Autodesk Fusion 360 part; units mm, degrees
note: some values were not read from the file. Set by a fixed rule: which face or edge a step refers to.
(part 3 of 3)
sketch "スケッチ8" plane through (0, 0, 2) normal (0, 0, 1) x (-1, 0, 0)
  line L0 (-93, 22) -> (-93, 18)
  line L1 (-93, 18) -> (-97, 18)
  line L2 (-97, 18) -> (-97, 22)
  line L3 (-97, 22) -> (-93, 22)
  line L4 (-13, 22) -> (-13, 18)
  line L5 (-13, 18) -> (-17, 18)
  line L6 (-17, 18) -> (-17, 22)
  line L7 (-17, 22) -> (-13, 22)
  line L8 (-47, -18) -> (-43, -18)
  line L9 (-43, -18) -> (-43, -22)
  line L10 (-43, -22) -> (-47, -22)
  line L11 (-47, -22) -> (-47, -18)
  line L12 (33, -18) -> (37, -18)
  line L13 (37, -18) -> (37, -22)
  line L14 (37, -22) -> (33, -22)
  line L15 (33, -22) -> (33, -18)
  arc A0 (-93.85, -22.9326) -> (-96.15, -22.9326) centre (-95, -20) ccw
  line L16 (-93.85, -22.9326) -> (-93.85, -24)
  line L17 (-93.85, -24) -> (-92, -24)
  line L18 (-92, -24) -> (-92, -27)
  line L19 (-92, -27) -> (-98, -27)
  line L20 (-98, -27) -> (-98, -24)
  line L21 (-98, -24) -> (-96.15, -24)
  line L22 (-96.15, -24) -> (-96.15, -22.9326)
  arc A1 (-73.85, -22.9326) -> (-76.15, -22.9326) centre (-75, -20) ccw
  line L23 (-73.85, -22.9326) -> (-73.85, -24)
  line L24 (-73.85, -24) -> (-72, -24)
  line L25 (-72, -24) -> (-72, -27)
  line L26 (-72, -27) -> (-78, -27)
  line L27 (-78, -27) -> (-78, -24)
  line L28 (-78, -24) -> (-76.15, -24)
  line L29 (-76.15, -24) -> (-76.15, -22.9326)
  arc A2 (-53.85, -22.9326) -> (-56.15, -22.9326) centre (-55, -20) ccw
  line L30 (-53.85, -22.9326) -> (-53.85, -24)
  line L31 (-53.85, -24) -> (-52, -24)
  line L32 (-52, -24) -> (-52, -27)
  line L33 (-52, -27) -> (-58, -27)
  line L34 (-58, -27) -> (-58, -24)
  line L35 (-58, -24) -> (-56.15, -24)
  line L36 (-56.15, -24) -> (-56.15, -22.9326)
  arc A3 (-33.85, -22.9326) -> (-36.15, -22.9326) centre (-35, -20) ccw
  line L37 (-33.85, -22.9326) -> (-33.85, -24)
  line L38 (-33.85, -24) -> (-32, -24)
  line L39 (-32, -24) -> (-32, -27)
  line L40 (-32, -27) -> (-38, -27)
  line L41 (-38, -27) -> (-38, -24)
  line L42 (-38, -24) -> (-36.15, -24)
  line L43 (-36.15, -24) -> (-36.15, -22.9326)
  arc A4 (-13.85, -22.9326) -> (-16.15, -22.9326) centre (-15, -20) ccw
  line L44 (-13.85, -22.9326) -> (-13.85, -24)
  line L45 (-13.85, -24) -> (-12, -24)
  line L46 (-12, -24) -> (-12, -27)
  line L47 (-12, -27) -> (-18, -27)
  line L48 (-18, -27) -> (-18, -24)
  line L49 (-18, -24) -> (-16.15, -24)
  line L50 (-16.15, -24) -> (-16.15, -22.9326)
  arc A5 (6.15, -22.9326) -> (3.85, -22.9326) centre (5, -20) ccw
  line L51 (6.15, -22.9326) -> (6.15, -24)
  line L52 (6.15, -24) -> (8, -24)
  line L53 (8, -24) -> (8, -27)
  line L54 (8, -27) -> (2, -27)
  line L55 (2, -27) -> (2, -24)
  line L56 (2, -24) -> (3.85, -24)
  line L57 (3.85, -24) -> (3.85, -22.9326)
  arc A6 (-18.85, -2.9326) -> (-21.15, -2.9326) centre (-20, 0) ccw
  line L58 (-18.85, -2.9326) -> (-18.85, -4)
  line L59 (-18.85, -4) -> (-17, -4)
  line L60 (-17, -4) -> (-17, -7)
  line L61 (-17, -7) -> (-23, -7)
  line L62 (-23, -7) -> (-23, -4)
  line L63 (-23, -4) -> (-21.15, -4)
  line L64 (-21.15, -4) -> (-21.15, -2.9326)
  arc A7 (26.15, -22.9326) -> (23.85, -22.9326) centre (25, -20) ccw
  line L65 (26.15, -22.9326) -> (26.15, -24)
  line L66 (26.15, -24) -> (28, -24)
  line L67 (28, -24) -> (28, -27)
  line L68 (28, -27) -> (22, -27)
  line L69 (22, -27) -> (22, -24)
  line L70 (22, -24) -> (23.85, -24)
  line L71 (23.85, -24) -> (23.85, -22.9326)
  arc A8 (46.15, -22.9326) -> (43.85, -22.9326) centre (45, -20) ccw
  line L72 (46.15, -22.9326) -> (46.15, -24)
  line L73 (46.15, -24) -> (48, -24)
  line L74 (48, -24) -> (48, -27)
  line L75 (48, -27) -> (42, -27)
  line L76 (42, -27) -> (42, -24)
  line L77 (42, -24) -> (43.85, -24)
  line L78 (43.85, -24) -> (43.85, -22.9326)
  arc A9 (66.15, -22.9326) -> (63.85, -22.9326) centre (65, -20) ccw
  line L79 (66.15, -22.9326) -> (66.15, -24)
  line L80 (66.15, -24) -> (68, -24)
  line L81 (68, -24) -> (68, -27)
  line L82 (68, -27) -> (62, -27)
  line L83 (62, -27) -> (62, -24)
  line L84 (62, -24) -> (63.85, -24)
  line L85 (63.85, -24) -> (63.85, -22.9326)
  arc A10 (86.15, -22.9326) -> (83.85, -22.9326) centre (85, -20) ccw
  line L86 (86.15, -22.9326) -> (86.15, -24)
  line L87 (86.15, -24) -> (88, -24)
  line L88 (88, -24) -> (88, -27)
  line L89 (88, -27) -> (82, -27)
  line L90 (82, -27) -> (82, -24)
  line L91 (82, -24) -> (83.85, -24)
  line L92 (83.85, -24) -> (83.85, -22.9326)
  arc A11 (81.15, -2.9326) -> (78.85, -2.9326) centre (80, 0) ccw
  line L93 (81.15, -2.9326) -> (81.15, -4)
  line L94 (81.15, -4) -> (83, -4)
  line L95 (83, -4) -> (83, -7)
  line L96 (83, -7) -> (77, -7)
  line L97 (77, -7) -> (77, -4)
  line L98 (77, -4) -> (78.85, -4)
  line L99 (78.85, -4) -> (78.85, -2.9326)
  arc A12 (61.15, -2.9326) -> (58.85, -2.9326) centre (60, 0) ccw
  line L100 (61.15, -2.9326) -> (61.15, -4)
  line L101 (61.15, -4) -> (63, -4)
  line L102 (63, -4) -> (63, -7)
  line L103 (63, -7) -> (57, -7)
  line L104 (57, -7) -> (57, -4)
  line L105 (57, -4) -> (58.85, -4)
  line L106 (58.85, -4) -> (58.85, -2.9326)
  arc A13 (41.15, -2.9326) -> (38.85, -2.9326) centre (40, 0) ccw
  line L107 (41.15, -2.9326) -> (41.15, -4)
  line L108 (41.15, -4) -> (43, -4)
  line L109 (43, -4) -> (43, -7)
  line L110 (43, -7) -> (37, -7)
  line L111 (37, -7) -> (37, -4)
  line L112 (37, -4) -> (38.85, -4)
  line L113 (38.85, -4) -> (38.85, -2.9326)
  arc A14 (21.15, -2.9326) -> (18.85, -2.9326) centre (20, 0) ccw
  line L114 (21.15, -2.9326) -> (21.15, -4)
  line L115 (21.15, -4) -> (23, -4)
  line L116 (23, -4) -> (23, -7)
  line L117 (23, -7) -> (17, -7)
  line L118 (17, -7) -> (17, -4)
  line L119 (17, -4) -> (18.85, -4)
  line L120 (18.85, -4) -> (18.85, -2.9326)
  arc A15 (1.15, -2.9326) -> (-1.15, -2.9326) centre (0, 0) ccw
  line L121 (1.15, -2.9326) -> (1.15, -4)
  line L122 (1.15, -4) -> (3, -4)
  line L123 (3, -4) -> (3, -7)
  line L124 (3, -7) -> (-3, -7)
  line L125 (-3, -7) -> (-3, -4)
  line L126 (-3, -4) -> (-1.15, -4)
  line L127 (-1.15, -4) -> (-1.15, -2.9326)
  arc A16 (-3.85, 17.0674) -> (-6.15, 17.0674) centre (-5, 20) ccw
  line L128 (-3.85, 17.0674) -> (-3.85, 16)
  line L129 (-3.85, 16) -> (-2, 16)
  line L130 (-2, 16) -> (-2, 13)
  line L131 (-2, 13) -> (-8, 13)
  line L132 (-8, 13) -> (-8, 16)
  line L133 (-8, 16) -> (-6.15, 16)
  line L134 (-6.15, 16) -> (-6.15, 17.0674)
  arc A17 (16.15, 17.0674) -> (13.85, 17.0674) centre (15, 20) ccw
  line L135 (16.15, 17.0674) -> (16.15, 16)
  line L136 (16.15, 16) -> (18, 16)
  line L137 (18, 16) -> (18, 13)
  line L138 (18, 13) -> (12, 13)
  line L139 (12, 13) -> (12, 16)
  line L140 (12, 16) -> (13.85, 16)
  line L141 (13.85, 16) -> (13.85, 17.0674)
  arc A18 (36.15, 17.0674) -> (33.85, 17.0674) centre (35, 20) ccw
  line L142 (36.15, 17.0674) -> (36.15, 16)
  line L143 (36.15, 16) -> (38, 16)
  line L144 (38, 16) -> (38, 13)
  line L145 (38, 13) -> (32, 13)
  line L146 (32, 13) -> (32, 16)
  line L147 (32, 16) -> (33.85, 16)
  line L148 (33.85, 16) -> (33.85, 17.0674)
  arc A19 (76.15, 17.0674) -> (73.85, 17.0674) centre (75, 20) ccw
  line L149 (76.15, 17.0674) -> (76.15, 16)
  line L150 (76.15, 16) -> (78, 16)
  line L151 (78, 16) -> (78, 13)
  line L152 (78, 13) -> (72, 13)
  line L153 (72, 13) -> (72, 16)
  line L154 (72, 16) -> (73.85, 16)
  line L155 (73.85, 16) -> (73.85, 17.0674)
  arc A20 (56.15, 17.0674) -> (53.85, 17.0674) centre (55, 20) ccw
  line L156 (56.15, 17.0674) -> (56.15, 16)
  line L157 (56.15, 16) -> (58, 16)
  line L158 (58, 16) -> (58, 13)
  line L159 (58, 13) -> (52, 13)
  line L160 (52, 13) -> (52, 16)
  line L161 (52, 16) -> (53.85, 16)
  line L162 (53.85, 16) -> (53.85, 17.0674)
  arc A21 (-38.85, -2.9326) -> (-41.15, -2.9326) centre (-40, 0) ccw
  line L163 (-38.85, -2.9326) -> (-38.85, -4)
  line L164 (-38.85, -4) -> (-37, -4)
  line L165 (-37, -4) -> (-37, -7)
  line L166 (-37, -7) -> (-43, -7)
  line L167 (-43, -7) -> (-43, -4)
  line L168 (-43, -4) -> (-41.15, -4)
  line L169 (-41.15, -4) -> (-41.15, -2.9326)
  arc A22 (-23.85, 17.0674) -> (-26.15, 17.0674) centre (-25, 20) ccw
  line L170 (-23.85, 17.0674) -> (-23.85, 16)
  line L171 (-23.85, 16) -> (-22, 16)
  line L172 (-22, 16) -> (-22, 13)
  line L173 (-22, 13) -> (-28, 13)
  line L174 (-28, 13) -> (-28, 16)
  line L175 (-28, 16) -> (-26.15, 16)
  line L176 (-26.15, 16) -> (-26.15, 17.0674)
  arc A23 (-43.85, 17.0674) -> (-46.15, 17.0674) centre (-45, 20) ccw
  line L177 (-43.85, 17.0674) -> (-43.85, 16)
  line L178 (-43.85, 16) -> (-42, 16)
  line L179 (-42, 16) -> (-42, 13)
  line L180 (-42, 13) -> (-48, 13)
  line L181 (-48, 13) -> (-48, 16)
  line L182 (-48, 16) -> (-46.15, 16)
  line L183 (-46.15, 16) -> (-46.15, 17.0674)
  arc A24 (-58.85, -2.9326) -> (-61.15, -2.9326) centre (-60, 0) ccw
  line L184 (-58.85, -2.9326) -> (-58.85, -4)
  line L185 (-58.85, -4) -> (-57, -4)
  line L186 (-57, -4) -> (-57, -7)
  line L187 (-57, -7) -> (-63, -7)
  line L188 (-63, -7) -> (-63, -4)
  line L189 (-63, -4) -> (-61.15, -4)
  line L190 (-61.15, -4) -> (-61.15, -2.9326)
  arc A25 (-78.85, -2.9326) -> (-81.15, -2.9326) centre (-80, 0) ccw
  line L191 (-78.85, -2.9326) -> (-78.85, -4)
  line L192 (-78.85, -4) -> (-77, -4)
  line L193 (-77, -4) -> (-77, -7)
  line L194 (-77, -7) -> (-83, -7)
  line L195 (-83, -7) -> (-83, -4)
  line L196 (-83, -4) -> (-81.15, -4)
  line L197 (-81.15, -4) -> (-81.15, -2.9326)
  line L198 (-53, 22) -> (-53, 18)
  line L199 (-53, 18) -> (-57, 18)
  line L200 (-57, 18) -> (-57, 22)
  line L201 (-57, 22) -> (-53, 22)
  line L202 (27, 22) -> (27, 18)
  line L203 (27, 18) -> (23, 18)
  line L204 (23, 18) -> (23, 22)
  line L205 (23, 22) -> (27, 22)
  line L206 (-7, -18) -> (-3, -18)
  line L207 (-3, -18) -> (-3, -22)
  line L208 (-3, -22) -> (-7, -22)
  line L209 (-7, -22) -> (-7, -18)
  line L210 (72, 2) -> (72, -2)
  line L211 (72, -2) -> (68, -2)
  line L212 (68, -2) -> (68, 2)
  line L213 (68, 2) -> (72, 2)
  line L214 (104, -37.5) -> (104, 37.5)
  line L215 (104, 37.5) -> (-104, 37.5)
  line L216 (-104, 37.5) -> (-104, -37.5)
  line L217 (-104, -37.5) -> (104, -37.5)
  line L218 (67, 22) -> (67, 18)
  line L219 (67, 18) -> (63, 18)
  line L220 (63, 18) -> (63, 22)
  line L221 (63, 22) -> (67, 22)
  line L222 (32, 2) -> (32, -2)
  line L223 (32, -2) -> (28, -2)
  line L224 (28, -2) -> (28, 2)
  line L225 (28, 2) -> (32, 2)
  line L226 (-48, 2) -> (-48, -2)
  line L227 (-48, -2) -> (-52, -2)
  line L228 (-52, -2) -> (-52, 2)
  line L229 (-52, 2) -> (-48, 2)
  line L230 (-88, 2) -> (-88, -2)
  line L231 (-88, -2) -> (-92, -2)
  line L232 (-92, -2) -> (-92, 2)
  line L233 (-92, 2) -> (-88, 2)
  line L234 (-8, 2) -> (-8, -2)
  line L235 (-8, -2) -> (-12, -2)
  line L236 (-12, -2) -> (-12, 2)
  line L237 (-12, 2) -> (-8, 2)
  line L238 (-87, -18) -> (-83, -18)
  line L239 (-83, -18) -> (-83, -22)
  line L240 (-83, -22) -> (-87, -22)
  line L241 (-87, -22) -> (-87, -18)
  line L242 (77, -18) -> (77, -22)
  line L243 (77, -22) -> (73, -22)
  line L244 (73, -22) -> (73, -18)
  line L245 (73, -18) -> (77, -18)
  circle A26 centre (98, -31.5) radius 4
  line L246 (104, 37.5) -> (104, -37.5)
  circle A27 centre (-98, -31.5) radius 4
  line L247 (-104, -37.5) -> (-104, 37.5)
  circle A28 centre (98, 30.5) radius 4
  circle A29 centre (-98, 30.5) radius 4
  dimension "d177" = 8
  dimension "d178" = 6
  dimension "d179" = 6
  dimension "d180" = 8
  dimension "d181" = 6
  dimension "d182" = 6
  dimension "d185" = 0
  dimension "d186" = 62
  measures "d168" distance of L21.end
  measures "d177" diameter of A26
  measures "d178" distance of L217 A26.centre
  measures "d179" distance of A26.centre L246
  measures "d180" diameter of A27
  measures "d181" distance of A27.centre L247
  measures "d182" distance of L217 A27.centre
extrude "押し出し7" cut sketch "スケッチ8" against normal up to surface (2 mm away) contours A26 | A27 | A28 | A29
